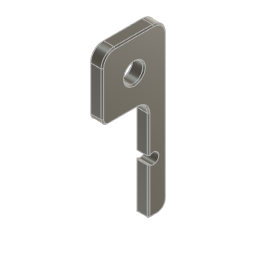
[a]_exhaust_filter_mount_x2 (Autodesk Fusion 360 design; units mm, degrees)
Autodesk Fusion 360 part; units mm, degrees
sketch "Sketch1" plane through (0, 0, 0) normal (1, 0, 0) x (0, 1, 0)
  line L0 (-12.6, 18.1567) -> (7.4, 18.1567)
  line L1 (7.4, 18.1567) -> (7.4, -33.3433)
  line L2 (7.4, -33.3433) -> (1.8, -33.3433)
  line L3 (1.8, -1.5933) -> (-12.6, -1.5933)
  line L4 (-12.6, -1.5933) -> (-12.6, 18.1567)
  circle A0 centre (-2.6, 8.1567) radius 3
  line L5 (7.4, 18.1567) -> (-2.6, 8.1567) construction
  line L6 (-12.6, 18.1567) -> (-2.6, 8.1567) construction
  arc A1 (1.8, -18.5433) -> (1.8, -16.9433) centre (3.3, -17.7433) ccw
  line L7 (1.8, -33.3433) -> (1.8, -18.5433)
  line L8 (1.8, -16.9433) -> (1.8, -1.5933)
  line L9 (2.244, -16.4933) -> (1.356, -16.4933)
  line L10 (1.356, -16.4933) -> (1.356, -18.9933)
  line L11 (1.356, -18.9933) -> (2.244, -18.9933)
  line L12 (2.244, -18.9933) -> (2.244, -16.4933)
  line L13 (2.244, -16.4933) -> (1.356, -18.9933) construction
  line L14 (1.356, -16.4933) -> (2.244, -18.9933) construction
  line L15 (3.3, -17.7433) -> (-0.8, -17.7433) construction
  point P0 (1.8, -17.7433)
  dimension "d1" = 20
  dimension "d2" = 19.75
  dimension "d3" = 6
  dimension "d4" = 45
  dimension "d5" = 45
  dimension "d6" = 5.6
  dimension "d7" = 3.4
  dimension "d8" = 15.6
  dimension "d10" = 1.5
  dimension "d24" = 31.75
  dimension "d25" = 8.1567
  dimension "d26" = 2.5
  constraint horizontal L0
  constraint perpendicular L0 L1
  constraint perpendicular L1 L2
  constraint perpendicular L2 L7
  constraint perpendicular L3 L7
  constraint perpendicular L0 L4
  constraint coincident A0.centre L5.end
  constraint coincident A1.end L7
  constraint collinear L7 L8
  constraint horizontal L9
  constraint perpendicular L9 L10
  constraint parallel L9 L11
  constraint parallel L10 L12
  constraint coincident L13 P0
  constraint coincident L14 P0
  constraint coincident A1.centre L15.start
  constraint perpendicular L12 L15
  constraint coincident P0 L15
  measures "d1" distance of L0.start L0.end
  measures "d2" distance of L0.start L3.end
  measures "d3" diameter of A0
  measures "d4" angle of L0 L5
  measures "d5" angle of L0 L6
  measures "d6" distance of L1.end L2.end
  measures "d7" diameter of A1
  measures "d8" distance of L2 A1.centre
  measures "d10" distance of A1.centre L8
  measures "d24" distance of L2 L3
  measures "d25" vertical distance of origin A0.centre
  measures "d26" distance of L9.end L10.end
extrude "Extrude1" add sketch "Sketch1" along normal mid plane 4 contours L0 L1 L2 L3 L4 A1 L7 L8 L9 L11
fillet "Fillet1" radius 4 2 edges at (0, -12.6, 18.1567) (0, 7.4, 18.1567)
fillet "Fillet2" radius 2 1 edges at (0, -12.6, -1.5933)
fillet "Fillet3" radius 3.4 1 edges at (0, 1.8, -1.5933)
fillet "Fillet4" radius 0.4 1 edges at (0, 1.8, -33.3433)
fillet "Fillet5" radius 3 1 edges at (0, 7.4, -33.3433)
chamfer "Chamfer1" distance 0.4 angle 45 28 edges at (2, -2.6, 18.1567) (2, -11.4284, 16.9851) (2, -12.6, 7.2817) (2, -12.0142, -1.0075) (2, -6.1, -1.5933) (2, 0.8042, -2.5891) (2, 1.8, -10.7433) (2, 1.8, -25.9683) (2, 1.9172, -33.2261) (2, 3.3, -33.3433) (2, 6.5213, -32.4646) (2, 7.4, -8.0933) (2, 6.2284, 16.9851) (2, -5.397, 9.2416) (-2, -2.6, 18.1567) (-2, 6.2284, 16.9851) (-2, 7.4, -8.0933) (-2, 6.5213, -32.4646) (-2, 3.3, -33.3433) (-2, 1.9172, -33.2261) (-2, 1.8, -25.9683) (-2, 1.8, -10.7433) (-2, 0.8042, -2.5891) (-2, -6.1, -1.5933) (-2, -12.0142, -1.0075) (-2, -12.6, 7.2817) (-2, -11.4284, 16.9851) (-2, -5.397, 7.0719)
